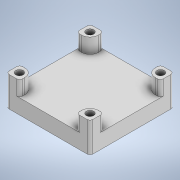
# Autodesk Inventor part: duzy_silnik_tyl
Saved by Autodesk Inventor 2020.3 (Build 243373000, 373)
## iProperties
Created: 2021-03-12
Part Number: duzy_silnik_tyl
Material: Generic
Document SubType Name: Modeling
Designer: patry
Density: 1 g/cm^3
Appearance: Default
Author: patry
Autodesk Inventor part; units mm, degrees
ref_plane "YZ Plane" through (0, 0, 0) normal (1, 0, 0) x (0, 1, 0)
ref_plane "XZ Plane" through (0, 0, 0) normal (0, 1, 0) x (-1, 0, 0)
ref_plane "XY Plane" through (0, 0, 0) normal (0, 0, 1) x (1, 0, 0)
sketch "Sketch1" plane through (0, 0, 0) normal (0, 1, 0) x (-1, 0, 0)
  line L0 (140, 0) -> (74, 0)
  line L1 (74, 0) -> (76, 0)
  line L2 (140, 0) -> (140, -60)
  line L3 (140, -60) -> (140, 0)
  line L4 (138, -58) -> (82, -2)
  line L5 (82, -58) -> (138, -2)
  circle A0 centre (110, -30) radius 19.4
  circle A1 centre (104, -30) radius 19.4
  line L6 (110, -30) -> (110, -49.4)
  line L7 (86.45, -6.45) -> (86.45, -53.55)
  line L8 (82, -58) -> (82, -2)
  line L9 (76, -58) -> (76, -2)
  line L10 (74, 0) -> (74, -60)
  line L11 (74, 0) -> (74, -60)
  circle A2 centre (86.45, -6.45) radius 2.5
  line L12 (76, -2) -> (138, -2)
  line L13 (80.45, -8.95) -> (133.55, -8.95)
  line L14 (80.45, -3.95) -> (133.55, -3.95)
  line L15 (133.55, -6.45) -> (86.45, -6.45)
  line L16 (82, -2) -> (138, -2)
  line L17 (104, -10.6) -> (110, -10.6)
  line L18 (138, -2) -> (138, -58)
  line L19 (138, -2) -> (138, -58)
  line L20 (133.55, -53.55) -> (133.55, -6.45)
  line L21 (140, -60) -> (138, -60)
  line L22 (138, -60) -> (138, -58)
  line L23 (138, -58) -> (140, -58)
  line L24 (140, -58) -> (140, -60)
  line L25 (104, -49.4) -> (110, -49.4)
  circle A3 centre (86.45, -53.55) radius 2.5
  line L26 (133.55, -51.05) -> (80.45, -51.05)
  line L27 (86.45, -53.55) -> (133.55, -53.55)
  line L28 (80.45, -56.05) -> (133.55, -56.05)
  line L29 (138, -58) -> (82, -58)
  line L30 (138, -58) -> (76, -58)
  line L31 (74, -60) -> (140, -60)
  line L32 (140, -60) -> (32, -60)
  circle A4 centre (127.55, -53.55) radius 2.5
  line L33 (104, -30) -> (104, -49.4)
  circle A5 centre (80.45, -6.45) radius 2.5
  line L34 (86.45, -53.55) -> (82, -53.55)
  line L35 (82, -58) -> (86.45, -58)
  line L36 (86.45, -58) -> (86.45, -53.55)
  line L37 (82, -53.55) -> (82, -58)
  circle A6 centre (80.45, -53.55) radius 2.5
  circle A7 centre (133.55, -53.55) radius 2.5
  line L38 (76, 0) -> (76, -2)
  line L39 (76, -2) -> (74, -2)
  line L40 (74, -2) -> (74, 0)
  line L41 (138, -2) -> (133.55, -2)
  line L42 (133.55, -2) -> (133.55, -6.45)
  line L43 (133.55, -6.45) -> (138, -6.45)
  line L44 (138, -6.45) -> (138, -2)
  circle A8 centre (127.55, -6.45) radius 2.5
  circle A9 centre (133.55, -6.45) radius 2.5
  line L45 (0, -25) -> (0, 0)
  line L46 (32, -60) -> (0, -25)
  line L47 (0, -25) -> (0, 0)
  line L48 (0, 0) -> (74, 0)
  line L49 (0, 0) -> (74, 0)
  line L50 (140, -60) -> (140, 0)
  line L51 (140, -60) -> (0, -60)
  line L52 (0, -60) -> (0, 0)
  line L53 (0, 0) -> (140, 0)
  line L54 (140, 0) -> (140, -60)
  line L55 (0, -60) -> (40, -60)
  line L56 (40, -60) -> (40, -100)
  line L57 (40, -100) -> (0, -100)
  line L58 (0, -100) -> (0, -60)
  line L59 (138, -58) -> (128.5, -58)
  line L60 (128.5, -58) -> (128.5, -48.5)
  line L61 (128.5, -48.5) -> (138, -48.5)
  line L62 (138, -48.5) -> (138, -58)
  line L63 (82, -58) -> (91.5, -58)
  line L64 (91.5, -58) -> (91.5, -48.5)
  line L65 (91.5, -48.5) -> (82, -48.5)
  line L66 (82, -48.5) -> (82, -58)
  line L67 (138, -2) -> (128.5, -2)
  line L68 (128.5, -2) -> (128.5, -11.5)
  line L69 (128.5, -11.5) -> (138, -11.5)
  line L70 (138, -11.5) -> (138, -2)
  line L71 (82, -2) -> (91.5, -2)
  line L72 (91.5, -2) -> (91.5, -11.5)
  line L73 (91.5, -11.5) -> (82, -11.5)
  line L74 (82, -11.5) -> (82, -2)
  point P0 (127.55, 3.95)
  point P1 (127.55, 8.95)
  point P2 (86.45, 3.95)
  point P3 (86.45, 8.95)
  point P4 (127.55, 56.05)
  point P5 (127.55, 51.05)
  point P6 (86.45, 56.05)
  point P7 (86.45, 51.05)
  point P8 (123.7179, -16.2821)
  point P9 (131.05, -8.95)
  point P10 (88.95, -8.95)
  point P11 (88.2178, -8.2178)
  point P12 (86.45, -8.95)
  point P13 (82, -3.95)
  point P14 (135.3178, -55.3178)
  point P15 (127.55, -56.05)
  point P16 (127.55, -51.05)
  point P17 (131.05, -51.05)
  point P18 (123.7179, -43.7179)
  point P19 (86.45, -51.05)
  point P20 (86.45, -56.05)
  point P21 (86.45, -3.95)
  point P22 (127.55, -8.95)
  point P23 (127.55, -3.95)
  point P24 (86.45, -8.95)
  point P25 (86.45, -3.95)
  point P26 (127.55, -56.05)
  point P27 (127.55, -51.05)
  point P28 (127.55, -8.95)
  point P29 (127.55, -3.95)
  point P30 (86.45, -51.05)
  point P31 (86.45, -56.05)
  dimension "d0" = 40
  dimension "d1" = 40
  dimension "d2" = 9.5
  dimension "d3" = 9.5
  dimension "d4" = 9.5
  dimension "d5" = 9.5
  dimension "d6" = 9.5
  dimension "d7" = 9.5
  dimension "d8" = 9.5
  dimension "d9" = 9.5
  constraints: 150 end point, 13 equal length, 12 point on circle, 10 centre point, 7 horizontal, 7 perpendicular, 5 point on line, 1 coincident
  measures "d0" distance of L56.end L57.end
  measures "d1" distance of L55.end L56.end
  measures "d2" distance of L60.end L61.end
  measures "d3" distance of L59.end L60.end
  measures "d4" distance of L65.end L64.end
  measures "d5" distance of L64.end L63.end
  measures "d6" distance of L69.end L68.end
  measures "d7" distance of L68.end L67.end
  measures "d8" distance of L72.end L73.end
  measures "d9" distance of L71.end L72.end
extrude "Extrusion1" add sketch "Sketch1" along normal blind 10 contours L29 L60 L28 A7 L4 | L4 A7 L20 L61 L18 | L12 L72 L14 L4 | L4 L14 L8 | A7 L27 L4 | L4 L20 A7 | L61 L20 L69 L18 | L29 L64 L28 L60 | L8 L28 L5 | L5 L28 L36 L29 | L14 A2 L4 | L4 A2 L13 L8 A5 L14 | L12 L68 L14 L72 | L27 A7 L4 | L4 A7 L20 | L28 L60 A4 L27 A7 | L69 L20 A9 L43 L18 | L61 L4 A0 L5 L69 L20 | L20 L26 L4 L61 | L29 L36 L28 L64 | L28 A4 L60 | L28 L8 A6 L34 A3 L5 | L5 A3 L28 | A2 L15 L4 | L4 L7 A2 | L14 L72 L15 A2 | A5 L8 | L12 L42 L14 L68 | L14 A8 L15 L72 | A7 L27 A4 L60 L26 L4 | L4 L26 A7 | L43 A9 L5 L18 | L69 L5 L13 L20 | L60 L26 L64 L5 A1 L25 A0 L4 | L4 L26 L60 | L64 L27 A4 L28 | L28 A3 L27 L64 | A4 L27 L60 | L60 L27 A4 | A3 L34 L5 | L5 L36 A3 | L36 L27 A3 | L8 L34 A6 | L15 A2 L4 | L4 A2 L7 | L13 L4 L73 L7 | L7 L73 L8 L13 | A2 L4 L13 | L15 L72 L13 L4 A2 | L12 L5 A9 L42 | L68 A8 L14 | L14 A9 L15 A8 L68 | A8 L68 L15 | L15 A8 L13 L72 | L27 L60 A4 | A9 L20 L43 | L43 L5 A9 | A9 L5 L20 | L13 L5 A9 | L68 L13 L5 | L5 A0 L17 A1 L4 L72 L13 L68 | A0 L6 A1 L4 | L4 A1 L5 A0 | L60 A4 L26 | L64 L26 A4 L27 | L27 A3 L5 L26 L64 | A4 L60 L27 | L7 A3 L5 | L34 A3 L7 | L5 A3 L27 | L34 A6 L8 L26 A3 | L8 A6 L34 | L73 L4 A1 L7 | L7 A1 L65 L8 L73 | L13 L72 L4 | A9 L5 L42 | L42 L15 A9 | A8 L15 L68 | L15 L68 A8 | L5 A9 L15 | L13 L68 A8 L15 A9 L5 | L5 A1 A0 | L13 A8 L68 | A1 L6 L4 | L4 L5 A1 | L25 A1 A0 | A0 A1 L6 | L26 L5 L64 | A3 L26 L5 | L26 L8 L65 L7 | L7 L65 L5 L26 | L7 A1 | A1 L4 A0 L5 L7 | A8 L68 L15 | L5 L4 A0 A1 | A0 A1 L17 | L5 A0 L4 | L6 A1 A0 L33 L5 | A1 L33 A0 | A1 L5 A0 L33 | L65 L7 A1 L5 | A1 A0 L4 | L33 A0 L5 picked at (82.1331, -6.9717)
sketch "Sketch2" plane through (0, 10, 0) normal (0, 1, 0) x (1, 0, 0)
  line L0 (-82, 58) -> (-138, 58) projected
  line L1 (-138, 2) -> (-82, 2) projected
  line L2 (-138, 58) -> (-82, 58)
  line L3 (-82, 58) -> (-82, 2)
  line L4 (-82, 2) -> (-138, 2)
  line L5 (-138, 2) -> (-138, 58)
  line L6 (-138, 58) -> (-138, 2) projected
  line L7 (-138, 58) -> (-129, 58)
  line L8 (-129, 58) -> (-129, 49)
  line L9 (-129, 49) -> (-138, 49)
  line L10 (-138, 49) -> (-138, 58)
  line L11 (-82, 58) -> (-91, 58)
  line L12 (-91, 58) -> (-91, 49)
  line L13 (-91, 49) -> (-82, 49)
  line L14 (-82, 49) -> (-82, 58)
  line L15 (-138, 2) -> (-129, 2)
  line L16 (-129, 2) -> (-129, 11)
  line L17 (-129, 11) -> (-138, 11)
  line L18 (-138, 11) -> (-138, 2)
  line L19 (-82, 2) -> (-91, 2)
  line L20 (-91, 2) -> (-91, 11)
  line L21 (-91, 11) -> (-82, 11)
  line L22 (-82, 11) -> (-82, 2)
  line L23 (-140, 0) -> (-74, 0)
  line L24 (-74, 0) -> (-76, 0)
  line L25 (-140, 0) -> (-140, 60)
  line L26 (-140, 60) -> (-140, 0)
  line L27 (-138, 58) -> (-82, 2)
  line L28 (-82, 58) -> (-138, 2)
  circle A0 centre (-110, 30) radius 19.4
  circle A1 centre (-104, 30) radius 19.4
  line L29 (-110, 30) -> (-110, 49.4)
  line L30 (-86.45, 6.45) -> (-86.45, 53.55)
  line L31 (-82, 58) -> (-82, 2)
  line L32 (-76, 58) -> (-76, 2)
  line L33 (-74, 0) -> (-74, 60)
  line L34 (-74, 0) -> (-74, 60)
  circle A2 centre (-86.45, 6.45) radius 2.5
  line L35 (-76, 2) -> (-138, 2)
  line L36 (-80.45, 8.95) -> (-133.55, 8.95)
  line L37 (-80.45, 3.95) -> (-133.55, 3.95)
  line L38 (-133.55, 6.45) -> (-86.45, 6.45)
  line L39 (-82, 2) -> (-138, 2)
  line L40 (-104, 10.6) -> (-110, 10.6)
  line L41 (-138, 2) -> (-138, 58)
  line L42 (-138, 2) -> (-138, 58)
  line L43 (-133.55, 53.55) -> (-133.55, 6.45)
  line L44 (-140, 60) -> (-138, 60)
  line L45 (-138, 60) -> (-138, 58)
  line L46 (-138, 58) -> (-140, 58)
  line L47 (-140, 58) -> (-140, 60)
  line L48 (-104, 49.4) -> (-110, 49.4)
  circle A3 centre (-86.45, 53.55) radius 2.5
  line L49 (-133.55, 51.05) -> (-80.45, 51.05)
  line L50 (-86.45, 53.55) -> (-133.55, 53.55)
  line L51 (-80.45, 56.05) -> (-133.55, 56.05)
  line L52 (-138, 58) -> (-82, 58)
  line L53 (-138, 58) -> (-76, 58)
  line L54 (-74, 60) -> (-140, 60)
  line L55 (-140, 60) -> (-32, 60)
  circle A4 centre (-127.55, 53.55) radius 2.5
  line L56 (-104, 30) -> (-104, 49.4)
  circle A5 centre (-80.45, 6.45) radius 2.5
  line L57 (-86.45, 53.55) -> (-82, 53.55)
  line L58 (-82, 58) -> (-86.45, 58)
  line L59 (-86.45, 58) -> (-86.45, 53.55)
  line L60 (-82, 53.55) -> (-82, 58)
  circle A6 centre (-80.45, 53.55) radius 2.5
  circle A7 centre (-133.55, 53.55) radius 2.5
  line L61 (-76, 0) -> (-76, 2)
  line L62 (-76, 2) -> (-74, 2)
  line L63 (-74, 2) -> (-74, 0)
  line L64 (-138, 2) -> (-133.55, 2)
  line L65 (-133.55, 2) -> (-133.55, 6.45)
  line L66 (-133.55, 6.45) -> (-138, 6.45)
  line L67 (-138, 6.45) -> (-138, 2)
  circle A8 centre (-127.55, 6.45) radius 2.5
  circle A9 centre (-133.55, 6.45) radius 2.5
  line L68 (0, 25) -> (0, 0)
  line L69 (-32, 60) -> (0, 25)
  line L70 (0, 25) -> (0, 0)
  line L71 (0, 0) -> (-74, 0)
  line L72 (0, 0) -> (-74, 0)
  line L73 (-140, 60) -> (-140, 0)
  line L74 (-140, 60) -> (0, 60)
  line L75 (0, 60) -> (0, 0)
  line L76 (0, 0) -> (-140, 0)
  line L77 (-140, 0) -> (-140, 60)
  line L78 (0, 60) -> (-40, 60)
  line L79 (-40, 60) -> (-40, 100)
  line L80 (-40, 100) -> (0, 100)
  line L81 (0, 100) -> (0, 60)
  line L82 (-138, 58) -> (-128.5, 58)
  line L83 (-128.5, 58) -> (-128.5, 48.5)
  line L84 (-128.5, 48.5) -> (-138, 48.5)
  line L85 (-138, 48.5) -> (-138, 58)
  line L86 (-82, 58) -> (-91.5, 58)
  line L87 (-91.5, 58) -> (-91.5, 48.5)
  line L88 (-91.5, 48.5) -> (-82, 48.5)
  line L89 (-82, 48.5) -> (-82, 58)
  line L90 (-138, 2) -> (-128.5, 2)
  line L91 (-128.5, 2) -> (-128.5, 11.5)
  line L92 (-128.5, 11.5) -> (-138, 11.5)
  line L93 (-138, 11.5) -> (-138, 2)
  line L94 (-82, 2) -> (-91.5, 2)
  line L95 (-91.5, 2) -> (-91.5, 11.5)
  line L96 (-91.5, 11.5) -> (-82, 11.5)
  line L97 (-82, 11.5) -> (-82, 2)
  point P0 (127.55, 3.95)
  point P1 (127.55, 8.95)
  point P2 (86.45, 3.95)
  point P3 (86.45, 8.95)
  point P4 (127.55, 56.05)
  point P5 (127.55, 51.05)
  point P6 (86.45, 56.05)
  point P7 (86.45, 51.05)
  point P8 (123.7179, -16.2821)
  point P9 (131.05, -8.95)
  point P10 (88.95, -8.95)
  point P11 (88.2178, -8.2178)
  point P12 (86.45, -8.95)
  point P13 (82, -3.95)
  point P14 (82, -2)
  point P15 (74, -2)
  point P16 (138, -60)
  point P17 (135.3178, -55.3178)
  point P18 (127.55, -56.05)
  point P19 (127.55, -51.05)
  point P20 (131.05, -51.05)
  point P21 (123.7179, -43.7179)
  point P22 (86.45, -51.05)
  point P23 (86.45, -56.05)
  point P24 (86.45, -3.95)
  point P25 (127.55, -8.95)
  point P26 (127.55, -3.95)
  point P27 (0, -25)
  point P28 (40, -60)
  point P29 (86.45, -8.95)
  point P30 (86.45, -3.95)
  point P31 (127.55, -56.05)
  point P32 (127.55, -51.05)
  point P33 (127.55, -8.95)
  point P34 (127.55, -3.95)
  point P35 (0, -25)
  point P36 (40, -60)
  point P37 (138, -60)
  point P38 (86.45, -51.05)
  point P39 (86.45, -56.05)
  point P40 (82, -2)
  point P41 (-91, 2)
  point P42 (-82, 11)
  point P43 (-138, 11)
  point P44 (-129, 2)
  dimension "d12" = 9
  dimension "d13" = 9
  dimension "d14" = 9
  dimension "d15" = 9
  dimension "d16" = 9
  dimension "d17" = 9
  dimension "d18" = 9
  dimension "d19" = 9
  dimension "d20" = 40
  dimension "d21" = 40
  dimension "d22" = 9.5
  dimension "d23" = 9.5
  dimension "d24" = 9.5
  dimension "d25" = 9.5
  dimension "d26" = 9.5
  dimension "d27" = 9.5
  dimension "d28" = 9.5
  dimension "d29" = 9.5
  constraints: 190 end point, 23 equal length, 12 perpendicular, 12 point on circle, 10 centre point, 5 horizontal, 5 point on line, 1 coincident
  measures "d12" distance of L8.end L9.end
  measures "d13" distance of L7.end L8.end
  measures "d14" distance of L13.end L12.end
  measures "d15" distance of L12.end L11.end
  measures "d16" distance of L17.end L16.end
  measures "d17" distance of L16.end L15.end
  measures "d18" distance of L20.end L21.end
  measures "d19" distance of L19.end L20.end
  measures "d20" distance of L79.end L80.end
  measures "d21" distance of L78.end L79.end
  measures "d22" distance of L83.end L84.end
  measures "d23" distance of L82.end L83.end
  measures "d24" distance of L88.end L87.end
  measures "d25" distance of L87.end L86.end
  measures "d26" distance of L92.end L91.end
  measures "d27" distance of L91.end L90.end
  measures "d28" distance of L95.end L96.end
  measures "d29" distance of L94.end L95.end
extrude "Extrusion2" add sketch "Sketch2" along normal blind 10 contours L28 L51 L59 L0 | L3 L51 L28 | L59 L51 L12 L0 | L3 A6 L57 A3 L28 L51 | L28 A3 L51 | A3 L50 L12 L51 | L3 L57 A6 | A3 L28 L49 L12 L50 | L3 A6 L57 | A6 L3 L49 A3 L57 | L27 L37 L3 | L1 L20 L37 L27 | A3 L49 L28 | L49 L3 L13 L30 | L30 L13 L28 L49 | L37 L27 A2 L36 L3 A5 | L37 A2 L27 | L8 L51 A7 L27 L0 | L49 L28 L12 | L20 L38 A2 L37 | A5 L3 | L27 A7 L43 L9 L5 | L8 A4 L50 A7 L51 | L20 L36 L27 A2 L38 | L8 L50 A4 | L1 L65 L37 L16 | L20 L27 L36 | L36 L30 L21 L3 | L27 L36 A2 | L36 L27 L21 L30 | L43 L49 L27 L9 | A7 L27 L49 | L8 A4 L50 | A4 L8 L49 L27 A7 L50 | L1 L28 A9 L65 | L37 A9 L38 A8 L16 | L27 L49 L8 | L5 L66 A9 L28 | A8 L38 L16 | L17 L43 A9 L66 L5 | A9 L28 L36 L16 A8 L38 | L38 A8 L16 | L17 L28 L36 L43 | A9 L36 L28 | L36 L28 L16 picked at (-82.2333, 6.0868)
fillet "Fillet1" radius 5.5 4 edges at (-91, 15, -49) (-129, 15, -49) (-129, 15, -11) (-91, 15, -11)
fillet "Fillet2" radius 2 12 edges at (-82, 10, -2) (-138, 10, -2) (-138, 10, -58) (-82, 10, -58) (-91, 15, -58) (-82, 15, -49) (-129, 15, -58) (-138, 15, -49) (-138, 15, -11) (-129, 15, -2) (-91, 15, -2) (-82, 15, -11)
sketch "Sketch3" plane through (0, 20, 0) normal (0, 1, 0) x (1, 0, 0)
  circle A0 centre (-133.55, 53.55) radius 2.5 projected
  circle A1 centre (-133.55, 53.55) radius 2.5
  circle A2 centre (-86.45, 53.55) radius 2.5 projected
  circle A3 centre (-86.45, 53.55) radius 2.5
  circle A4 centre (-133.55, 6.45) radius 2.5 projected
  circle A5 centre (-133.55, 6.45) radius 2.5
  circle A6 centre (-86.45, 6.45) radius 2.5 projected
  circle A7 centre (-86.45, 6.45) radius 2.5
  point P0 (0, 0)
  constraints: 4 centre point, 4 coincident
extrude "Extrusion3" cut sketch "Sketch3" against normal through all
body "Solid1"
